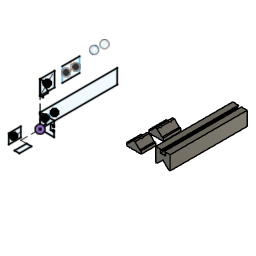
Rail additional version (Autodesk Fusion 360 design; units mm, degrees)
Autodesk Fusion 360 part; units mm, degrees
sketch "스케치1" plane through (0, 0, 0) normal (1, 0, 0) x (0, 1, 0)
  line L0 (15, 7.5) -> (5, 7.5) construction
  line L1 (15.072, 8.9983) -> (5.072, 8.9983)
  line L2 (15.0158, 6.0001) -> (5.0113, 6)
  line L3 (0, 0) -> (80, 0)
  line L4 (80, 0) -> (80, 15)
  line L5 (80, 15) -> (0, 15)
  line L6 (0, 15) -> (0, 0)
  arc A0 (15.0158, 6.0001) -> (15.072, 8.9983) centre (15, 7.5) ccw
  arc A1 (5.072, 8.9983) -> (5.0113, 6) centre (5, 7.5) ccw
  line L7 (0, 0) -> (0, 30) construction
  line L8 (0, 30) -> (15, 30)
  line L9 (15, 30) -> (15, 45)
  line L10 (15, 45) -> (0, 45)
  line L11 (0, 45) -> (0, 30)
  line L12 (0, 30) -> (15, 45) construction
  circle A2 centre (7.5, 37.5) radius 1.5
  line L13 (23.013, 45) -> (41.013, 45)
  line L14 (41.013, 45) -> (41.013, 30)
  line L15 (41.013, 30) -> (23.013, 30)
  line L16 (23.013, 30) -> (23.013, 45)
  line L17 (23.013, 37.5) -> (41.013, 37.5) construction
  circle A3 centre (27.013, 37.5) radius 1.5
  circle A4 centre (37.013, 37.5) radius 1.5
  line L18 (32.013, 45) -> (32.013, 30) construction
  line L19 (-20, 12.5) -> (-32.5, 12.5)
  line L20 (-32.5, 12.5) -> (-32.5, 2.5)
  line L21 (-32.5, 2.5) -> (-20, 2.5)
  line L22 (-20, 2.5) -> (-20, 12.5)
  circle A5 centre (-27.5, 7.5) radius 1.5
  line L23 (-27.5, 7.5) -> (-20, 7.5) construction
  circle A6 centre (56.1257, 43.1349) radius 2.7 construction
  line L24 (54.5669, 45.8349) -> (57.6846, 45.8349)
  line L25 (57.6846, 45.8349) -> (59.2434, 43.1349)
  line L26 (59.2434, 43.1349) -> (57.6846, 40.4349)
  line L27 (57.6846, 40.4349) -> (54.5669, 40.4349)
  line L28 (54.5669, 40.4349) -> (53.008, 43.1349)
  line L29 (53.008, 43.1349) -> (54.5669, 45.8349)
  circle A7 centre (66.8412, 42.9043) radius 1.5
  dimension "d15" = 15
  dimension "d16" = 10
  dimension "d21" = 1.5
  dimension "d22" = 80
  dimension "d23" = 5
  dimension "d24" = 1.5
  dimension "d33" = 30
  dimension "d34" = 3
  dimension "d35" = 18
  dimension "d36" = 3
  dimension "d37" = 10
  dimension "d56" = 10
  dimension "d58" = 12.5
  dimension "d59" = 3
  dimension "d60" = 7.5
  dimension "d61" = 20
  dimension "d63" = 5.4
  dimension "d64" = 120
  dimension "d65" = 120
  dimension "d66" = 3
  constraint horizontal L0
  constraint horizontal L3
  constraint vertical L4
  constraint horizontal L5
  constraint vertical L6
  constraint coincident L3.start L6.end
  constraint symmetric L0 L3 L5
  constraint horizontal L1
  constraint coincident L0.start A0.centre
  constraint coincident L0.end A1.centre
  constraint perpendicular L3 L7
  constraint horizontal L8
  constraint vertical L9
  constraint horizontal L10
  constraint vertical L11
  constraint equal L6 L8
  constraint equal L6 L11
  constraint midpoint L12 A2.centre
  constraint horizontal L13
  constraint vertical L14
  constraint horizontal L15
  constraint vertical L16
  constraint collinear L8 L15
  constraint collinear L10 L13
  constraint midpoint L16 L17.start
  constraint midpoint L14 L17.end
  constraint coincident L17 A3.centre
  constraint coincident L17 A4.centre
  constraint equal A3 A4
  constraint midpoint L13 L18.start
  constraint midpoint L15 L18.end
  constraint symmetric A3 A4 L18
  constraint horizontal L19
  constraint perpendicular L19 L20
  constraint perpendicular L20 L21
  constraint perpendicular L19 L22
  constraint symmetric L0 L19 L21
  constraint coincident A5.centre L23.start
  constraint midpoint L22 L23.end
  constraint horizontal L23
  constraint tangent A6 L24
  constraint tangent A6 L25
  constraint tangent A6 L26
  constraint tangent A6 L27
  constraint tangent A6 L28
  constraint tangent A6 L29
  constraint horizontal L24
  constraint horizontal L27
  constraint parallel L25 L28
  constraint parallel L26 L29
  measures "d15" distance of L3.start L5.end
  measures "d16" distance of L0.start L0.end
  measures "d21" radius of A0
  measures "d22" distance of L3.start L3.end
  measures "d23" distance of L0.end L6
  measures "d24" radius of A1
  measures "d33" distance of L3.start L7.end
  measures "d35" distance of L14.end L15.end
  measures "d36" diameter of A3
  measures "d37" distance of A3.centre A4.centre
  measures "d56" distance of L19.end L20.end
  measures "d58" distance of L19.start L19.end
  measures "d59" diameter of A5
  measures "d60" distance of A5.centre L23.end
  measures "d61" distance of L6 L22
  measures "d63" diameter of A6
  measures "d64" angle of L24 L25
  measures "d65" angle of L25 L26
  measures "d66" diameter of A7
sketch "스케치2" plane through (0, 0, 0) normal (0, 1, 0) x (1, 0, 0)
  line L0 (0, 0) -> (0, -1.5)
  line L1 (0, -1.5) -> (6, -7.5)
  line L2 (6, -7.5) -> (0, -13.5)
  line L3 (0, -13.5) -> (0, -15)
  line L4 (0, -15) -> (14.5, -15)
  line L5 (14.5, -15) -> (14.5, -9)
  line L6 (14.5, -9) -> (13.5, -9)
  line L7 (13.5, -9) -> (13.5, -10.2)
  line L8 (13.5, -10.2) -> (11, -10.2)
  line L9 (11, -10.2) -> (11, -4.8)
  line L10 (11, -4.8) -> (13.5, -4.8)
  line L11 (13.5, -4.8) -> (13.5, -6)
  line L12 (13.5, -6) -> (14.5, -6)
  line L13 (14.5, -6) -> (14.5, 0)
  line L14 (14.5, 0) -> (0, 0)
  line L15 (0, -45) -> (3, -45)
  line L16 (3, -45) -> (3, -43.5)
  line L17 (3, -43.5) -> (8, -38.5)
  line L18 (8, -38.5) -> (8, -36.5)
  line L19 (8, -36.5) -> (3, -31.5)
  line L20 (3, -31.5) -> (3, -30)
  line L21 (3, -30) -> (0, -30)
  line L22 (0, -30) -> (0, -45)
  line L23 (0, 0) -> (0, -30) construction
  line L24 (13.5, -10.2) -> (14.5, -10.2)
  line L25 (13.5, -4.8) -> (14.5, -4.8)
  dimension "d6" = 5.4
  dimension "d7" = 1
  dimension "d8" = 3
  dimension "d9" = 135
  dimension "d10" = 135
  dimension "d11" = 5
  dimension "d12" = 2.5
  dimension "d13" = 6
  dimension "d14" = 6
  dimension "d25" = 135
  dimension "d26" = 2
  dimension "d27" = 135
  dimension "d28" = 5
  dimension "d29" = 15
  dimension "d31" = 3
  dimension "d32" = 30
  constraint vertical L0
  constraint vertical L3
  constraint perpendicular L3 L4
  constraint perpendicular L4 L5
  constraint perpendicular L5 L6
  constraint perpendicular L6 L7
  constraint perpendicular L7 L8
  constraint perpendicular L8 L9
  constraint perpendicular L9 L10
  constraint perpendicular L10 L11
  constraint perpendicular L11 L12
  constraint perpendicular L12 L13
  constraint perpendicular L0 L14
  constraint equal L5 L13
  constraint equal L7 L11
  constraint collinear L7 L11
  constraint collinear L5 L13
  constraint equal L0 L3
  constraint collinear L0 L3
  constraint horizontal L15
  constraint perpendicular L15 L16
  constraint parallel L16 L18
  constraint parallel L16 L20
  constraint perpendicular L16 L21
  constraint perpendicular L15 L22
  constraint equal L16 L20
  constraint collinear L16 L20
  constraint coincident L0.start L14.end
  constraint vertical L23
  constraint coincident L5 L24.end
  constraint perpendicular L5 L24
  constraint coincident L13 L25.end
  constraint perpendicular L13 L25
  measures "d6" distance of L8.end L9.end
  measures "d7" distance of L5.end L6.end
  measures "d8" distance of L6 L12
  measures "d9" angle of L2 L3
  measures "d10" angle of L0 L1
  measures "d11" distance of L1.end L9
  measures "d12" distance of L7.end L8.end
  measures "d13" distance of L12.end L13.end
  measures "d14" distance of L0 L1.end
  measures "d25" angle of L19 L20
  measures "d26" distance of L17.end L18.end
  measures "d27" angle of L16 L17
  measures "d28" distance of L18 L20
  measures "d29" distance of L15.start L21.end
  measures "d31" distance of L20.end L21.end
  measures "d32" distance of L21.end L0.start
extrude "돌출1" add sketch "스케치2" along normal blind 80 contours L0 L1 L2 L3 L4 L5 L8 L9 L10 L13 L14 L24 L25 | L11 L12 L13 L25 | L5 L6 L7 L24 makes body 1
extrude "돌출2" add sketch "스케치2" along normal blind 85 separate body contours L15 L16 L17 L18 L19 L20 L21 L22 makes body 2
extrude "돌출3" add sketch "스케치1" along normal blind 130 separate body contours L1 L2 A0 A1 makes body 3
extrude "돌출4" add sketch "스케치1" along normal blind 35 separate body contours L8 L9 L10 L11 makes body 4
extrude "돌출5" add sketch "스케치1" along normal blind 30 separate body contours L13 L14 L15 L16 makes body 5
combine "결합1" operation cut target body 1 tool bodies 3
combine "결합2" operation intersect target body 2 tool bodies 4
extrude "돌출6" add sketch "스케치2" along normal blind 55 separate body contours L15 L16 L17 L18 L19 L20 L21 L22 makes body 6
combine "결합3" operation intersect target body 5 tool bodies 6
pattern_linear "R-패턴1" count 4 spacing 20 along (0, 1, 0) of "결합1"
move_body "이동1" bodies 5 2 1 to x (0, 0, 1) y (0, 1, 0) z (-1, 0, 0) at (135, 0, 30)
sketch "스케치4" plane through (0, 0, 0) normal (0, 0, 1) x (1, 0, 0)
  line L0 (0, 0) -> (0, -20) construction
  line L1 (0, -20) -> (6, -20) construction
  line L2 (6, -20) -> (11, -20)
  line L3 (11, -20) -> (11, -32.5)
  line L4 (11, -32.5) -> (6, -32.5)
  line L5 (6, -32.5) -> (6, -20)
  dimension "d54" = 6
  dimension "d55" = 5
  dimension "d57" = 12.5
  dimension "d62" = 20
  constraint coincident L0.start origin
  constraint vertical L0
  constraint perpendicular L0 L1
  constraint horizontal L2
  constraint vertical L3
  constraint horizontal L4
  constraint vertical L5
  measures "d54" distance of L0.end L1.end
  measures "d55" distance of L3.end L4.end
  measures "d57" distance of L2.end L3.end
  measures "d62" distance of L0.start L0.end
equation "m3nut_height = 2.5 mm"
equation "m3nut_width = 5.4 mm"
equation "m3hole = 3 mm"
equation "d6 = m3nut_width"
equation "d8 = m3hole"
equation "d12 = m3nut_height"
equation "d15 = d13 * 2 + d8"
equation "d21 = m3hole / 2"
equation "d23 = d16 / 2"
equation "d24 = m3hole / 2"
equation "d28 = d14 - d26 / 2"
equation "d29 = d8 + 2 * d13"
equation "d34 = m3hole"
equation "d36 = m3hole"
equation "d37 = d16"
equation "d54 = d14"
equation "d55 = d11"
equation "d57 = d56 / 2 + d29 / 2"
equation "d58 = d57"
equation "d59 = m3hole"
equation "d60 = d29 / 2"
equation "d62 = d61"
equation "d63 = m3nut_width"
equation "d66 = m3hole"
